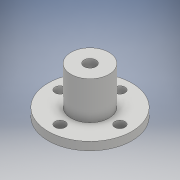
# Autodesk Inventor part: frange
Saved by Autodesk Inventor 2018 (Build 220112000, 112)
## iProperties
Created: 2019-03-10
Part Number: frange
Material: 一般
Document SubType Name: Modeling
Designer: ku_sk
Density: 1 g/cm^3
Appearance: 既定
Author: ku_sk
Autodesk Inventor part; units mm, degrees
ref_plane "YZ Plane" through (0, 0, 0) normal (1, 0, 0) x (0, 1, 0)
ref_plane "XZ Plane" through (0, 0, 0) normal (0, 1, 0) x (-1, 0, 0)
ref_plane "XY Plane" through (0, 0, 0) normal (0, 0, 1) x (1, 0, 0)
sketch "スケッチ1" plane through (0, 0, 0) normal (0, 0, 1) x (1, 0, 0)
  circle A0 centre (0, 0) radius 11
  dimension "d0" = 22
  constraints: 1 centre point, 1 coincident
  measures "d0" diameter of A0
extrude "押し出し1" add sketch "スケッチ1" along normal blind 2.16
sketch "スケッチ2" plane through (0, 0, 2.16) normal (0, 0, 1) x (1, 0, 0)
  circle A0 centre (0, 0) radius 5
  dimension "d3" = 10
  constraints: 1 centre point, 1 coincident
  measures "d3" diameter of A0
extrude "押し出し2" add sketch "スケッチ2" along normal blind 10
sketch "スケッチ3" plane through (0, 0, 12.16) normal (0, 0, 1) x (1, 0, 0)
  circle A0 centre (0, 0) radius 1.565
  dimension "d6" = 3.13
  constraints: 1 centre point, 1 coincident
  measures "d6" diameter of A0
extrude "押し出し3" cut sketch "スケッチ3" against normal up to surface (12.16 mm away)
sketch "スケッチ4" plane through (0, 0, 2.16) normal (0, 0, 1) x (1, 0, 0)
  circle A0 centre (0, 7.85) radius 1.35
  line L0 (0, -15.7768) -> (0, 17.6611) projected
  point P0 (0, 0)
  point P1 (0, 6.5)
  dimension "d9" = 2.7
  dimension "d10" = 6.5
  constraints: 2 point on line, 1 vertical alignment, 2 other
  measures "d10" distance of point (0, 0) point (0, 6.5)
extrude "押し出し4" cut sketch "スケッチ4" against normal up to surface (2.16 mm away)
pattern_circular "円形状パターン1" count 4 over 360 about axis through (0, 0, -10) along (0, 0, 1) of "押し出し4"
